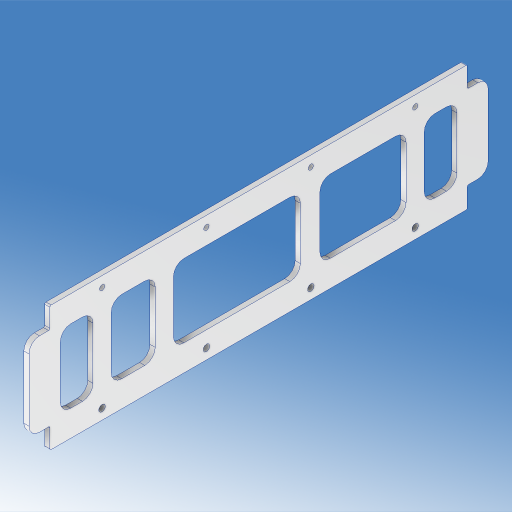
# Autodesk Inventor part: ChassisInterface
Saved by Autodesk Inventor 2024 (Build 280153000, 153)
## iProperties
Created: 2022-11-13
Part Number: ChassisInterface
Material: Aluminum 6061
Document SubType Name: Modeling
Designer: kumpu
Density: 2.7 g/cm^3
Appearance: Aluminum - Flat
Mass: 777.044 g
Surface Area: 1099.09 cm^2
Volume: 287.794 cm^3
Author: kumpu
Autodesk Inventor part; units mm, degrees
ref_plane "YZ Plane" through (0, 0, 0) normal (1, 0, 0) x (0, 1, 0)
ref_plane "XZ Plane" through (0, 0, 0) normal (0, 1, 0) x (-1, 0, 0)
ref_plane "XY Plane" through (0, 0, 0) normal (0, 0, 1) x (1, 0, 0)
sketch "Sketch1" plane through (0, 0, 0) normal (1, 0, 0) x (0, 1, 0)
  line L0 (76.2, 254) -> (-76.2, 254)
  line L1 (-76.2, 254) -> (-76.2, -254)
  line L2 (-76.2, -254) -> (76.2, -254)
  line L3 (76.2, -254) -> (76.2, 254)
  line L4 (76.2, 254) -> (-76.2, -254) construction
  line L5 (-76.2, 254) -> (76.2, -254) construction
  line L6 (50.8, 279.4) -> (-50.8, 279.4)
  line L7 (-50.8, 279.4) -> (-50.8, 254)
  line L8 (-50.8, 254) -> (50.8, 254)
  line L9 (50.8, 254) -> (50.8, 279.4)
  line L10 (50.8, 279.4) -> (-50.8, 254) construction
  line L11 (-50.8, 279.4) -> (50.8, 254) construction
  line L12 (50.8, -254) -> (-50.8, -254)
  line L13 (-50.8, -254) -> (-50.8, -279.4)
  line L14 (-50.8, -279.4) -> (50.8, -279.4)
  line L15 (50.8, -279.4) -> (50.8, -254)
  line L16 (50.8, -254) -> (-50.8, -279.4) construction
  line L17 (-50.8, -254) -> (50.8, -279.4) construction
  line L18 (0, 266.7) -> (0, -266.7) construction
  point P0 (0, 0)
  point P1 (-50.8, -254)
  point P2 (50.8, 254)
  dimension "d0" = 152.4
  dimension "d1" = 508
  dimension "d9" = 25.4
  dimension "d10" = 101.6
  constraints: 38 end point, 7 midpoint, 6 parallel, 3 horizontal, 3 perpendicular, 2 equal length, 1 point on line, 1 vertical
  measures "d0" distance of L2.end L1.end
  measures "d1" distance of L1.end L0.end
  measures "d9" distance of L14.end L12.start
  measures "d10" distance of L13.end L14.end
extrude "Extrusion1" add sketch "Sketch1" along normal mid plane 6.35
sketch "Sketch3" plane through (3.175, 0, 0) normal (1, 0, 0) x (0, 0, -1)
  line L0 (-241.3, 44.45) -> (-201.6125, 44.45)
  line L1 (-201.6125, 44.45) -> (-201.6125, -44.45)
  line L2 (-201.6125, -44.45) -> (-241.3, -44.45)
  line L3 (-241.3, -44.45) -> (-241.3, 44.45)
  line L4 (-179.3875, 44.45) -> (-125.857, 44.45)
  line L5 (-125.857, 44.45) -> (-125.857, -44.45)
  line L6 (-125.857, -44.45) -> (-179.3875, -44.45)
  line L7 (-179.3875, -44.45) -> (-179.3875, 44.45)
  line L8 (-103.632, 44.45) -> (50.8, 44.45)
  line L9 (50.8, 44.45) -> (50.8, -44.45)
  line L10 (50.8, -44.45) -> (-103.632, -44.45)
  line L11 (-103.632, -44.45) -> (-103.632, 44.45)
  line L12 (74.6125, 44.45) -> (179.3875, 44.45)
  line L13 (179.3875, 44.45) -> (179.3875, -44.45)
  line L14 (179.3875, -44.45) -> (74.6125, -44.45)
  line L15 (74.6125, -44.45) -> (74.6125, 44.45)
  line L16 (201.6125, -44.45) -> (241.3, -44.45)
  line L17 (241.3, -44.45) -> (241.3, 44.45)
  line L18 (241.3, 44.45) -> (201.6125, 44.45)
  line L19 (201.6125, 44.45) -> (201.6125, -44.45)
  line L20 (-201.6125, 0) -> (-179.3875, 0) construction
  line L21 (-125.857, 0) -> (-103.632, 0) construction
  line L22 (179.3875, 0) -> (201.6125, 0) construction
  line L23 (-254, -50.8) -> (-254, -76.2) construction
  circle A0 centre (-190.5, 63.5) radius 3.175
  line L24 (-190.5, 63.5) -> (-190.5, 0) construction
  line L25 (-190.5, 0) -> (-190.5, -63.5) construction
  circle A1 centre (-190.5, -63.5) radius 3.9751
  circle A2 centre (-63.5, 63.5) radius 3.175
  circle A3 centre (-63.5, -63.5) radius 3.9751
  circle A4 centre (63.5, 63.5) radius 3.175
  circle A5 centre (63.5, -63.5) radius 3.9751
  circle A6 centre (190.5, 63.5) radius 3.175
  circle A7 centre (190.5, -63.5) radius 3.9751
  line L26 (-125.857, 44.45) -> (-103.632, 44.45)
  line L27 (-103.632, 44.45) -> (-103.632, -44.45)
  line L28 (-103.632, -44.45) -> (-125.857, -44.45)
  line L29 (-125.857, -44.45) -> (-125.857, 44.45)
  line L30 (254, -76.2) -> (254, -50.8) projected
  line L31 (-254, -76.2) -> (254, -76.2) projected
  point P0 (0, 0)
  point P1 (0, 0)
  point P2 (-114.7445, 0)
  dimension "d12" = 22.225
  dimension "d13" = 12.7
  dimension "d14" = 88.9
  dimension "d16" = 6.35
  dimension "d17" = 7.9502
  dimension "d20" = 127
  dimension "d29" = 12.7
  dimension "d30" = 63.5
  dimension "d31" = 12.7
  dimension "d32" = 11.1125
  dimension "d33" = 31.75
  dimension "d34" = 127
  dimension "d35" = 63.5
  dimension "d39" = 154.432
  constraints: 58 end point, 12 parallel, 8 centre point, 8 midpoint, 7 collinear, 7 horizontal, 7 perpendicular, 4 point on line, 2 coincident, 1 vertical, 12 other
  measures "d12" distance of L20.start L20.end
  measures "d13" distance between parallel lines of L23 L3
  measures "d14" distance of L2.end L0.start
  measures "d16" diameter of A0
  measures "d17" diameter of A1
  measures "d20" distance of L24.start A2.centre
  measures "d29" distance from line of L9 A4.centre
  measures "d30" distance between parallel lines of L23 L25
  measures "d31" distance between parallel lines of L30 L17
  measures "d32" distance from line of A4.centre L15
  measures "d33" distance between parallel lines of L31 L2
  measures "d34" distance of L25.end L24.start
  measures "d35" distance from line of L20 L24.start
  measures "d39" distance between parallel lines of L9 L27
extrude "Extrusion3" cut sketch "Sketch3" against normal through all contours L0 L1 L2 L3 | L4 L5 L6 L7 | L8 L9 L10 L11 | L12 L13 L14 L15 | L19 L18 L17 L16 | A0 | A1 | A2 | A3 | A4 | A5 | A6 | A7
fillet "Fillet1" radius 12.7 24 edges at (0, 50.8, 279.4) (0, 44.45, 241.3) (0, 44.45, 201.6125) (0, -44.45, 201.6125) (0, -44.45, 241.3) (0, -50.8, 279.4) (0, -44.45, 179.3875) (0, 44.45, 179.3875) (0, -44.45, -50.8) (0, -44.45, -74.6125) (0, 44.45, -74.6125) (0, 44.45, -50.8) (0, 44.45, -179.3875) (0, 44.45, -201.6125) (0, 44.45, -241.3) (0, 50.8, -279.4) (0, -50.8, -279.4) (0, -44.45, -241.3) (0, -44.45, -201.6125) (0, -44.45, -179.3875) (0, 44.45, 125.857) (0, 44.45, 103.632) (0, -44.45, 103.632) (0, -44.45, 125.857)
fillet "Fillet1" radius 1.5875 8 edges at (0, 50.8, 254) (0, -50.8, 254) (0, -76.2, 254) (0, 76.2, 254) (0, 76.2, -254) (0, 50.8, -254) (0, -50.8, -254) (0, -76.2, -254)
sketch "Sketch4" plane through (-3.175, 0, 0) normal (-1, 0, 0) x (0, 0, 1)
  line L0 (-182.626, 63.5635) -> (-141.351, 63.5635) construction
  line L1 (-254, 74.6125) -> (-254, 52.3875) construction
  line L2 (252.4125, 76.2) -> (-252.4125, 76.2) construction
  point P0 (0, 0)
  dimension "d36" = 71.374
  dimension "d37" = 12.6365
  dimension "d38" = 41.275
  constraints: 2 end point, 1 horizontal
  measures "d36" distance from line of L1 L0.start
  measures "d37" distance between parallel lines of L2 L0
  measures "d38" distance of L0.start L0.end
body "Solid1"
